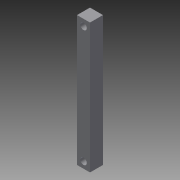
# Autodesk Inventor part: 5 in bar
Saved by Autodesk Inventor 2014 (Build 180170000, 170)
## iProperties
Created: 2014-01-31
Part Number: 5 in bar
Material: Generic
Document SubType Name: Modeling
Designer: Michael
Density: 1 g/cm^3
Appearance: Default
Author: Michael
Autodesk Inventor part; units mm, degrees
ref_plane "YZ Plane" through (0, 0, 0) normal (1, 0, 0) x (0, 1, 0)
ref_plane "XZ Plane" through (0, 0, 0) normal (0, 1, 0) x (-1, 0, 0)
ref_plane "XY Plane" through (0, 0, 0) normal (0, 0, 1) x (1, 0, 0)
sketch "Sketch1" plane through (0, 0, 0) normal (0, 0, 1) x (1, 0, 0)
  line L0 (-6.35, -63.5) -> (6.35, -63.5)
  line L1 (6.35, -63.5) -> (6.35, 63.5)
  line L2 (6.35, 63.5) -> (-6.35, 63.5)
  line L3 (-6.35, 63.5) -> (-6.35, -63.5)
  line L4 (-6.35, -63.5) -> (6.35, 63.5) construction
  line L5 (6.35, -63.5) -> (-6.35, 63.5) construction
  point P0 (0, 0)
  dimension "d0" = 12.7
  dimension "d1" = 127
  constraints: 12 end point, 2 midpoint, 2 parallel, 1 horizontal, 1 perpendicular
  measures "d0" distance of L2.end L1.end
  measures "d1" distance of L1.end L0.end
extrude "Extrusion1" add sketch "Sketch1" along normal blind 12.7
sketch "Sketch2" plane through (0, 0, 12.7) normal (0, 0, 1) x (1, 0, 0)
  line L0 (-6.35, -63.5) -> (6.35, -63.5) projected
  line L1 (6.35, 63.5) -> (-6.35, 63.5) projected
  line L2 (-6.35, 63.5) -> (-6.35, -63.5) projected
  line L3 (0, 63.5) -> (0, 57.15)
  line L4 (0, -63.5) -> (0, -57.15)
  point P0 (0, 0)
  dimension "d4" = 6.35
  dimension "d5" = 6.35
  constraints: 4 end point, 2 midpoint, 1 collinear, 1 parallel
  measures "d4" distance of L3.start L3.end
  measures "d5" distance of L4.start L4.end
hole "Hole1" at (0, 57.15, 12.7) at (0, -57.15, 12.7) direction (0, 0, -1) diameter 6.35 end through all
body "Solid1"
